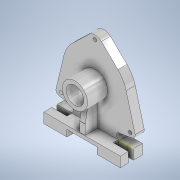
# Autodesk Inventor part: COMPRESSOR 1
Saved by Autodesk Inventor 2022 (Build 260153000, 153)
## iProperties
Created: 2023-06-16
Part Number: COMPRESSOR 1
Material: Aluminum 6061-AHC
Document SubType Name: Modeling
Designer: SENAI
Density: 2.7 g/cm^3
Appearance: Aluminum - Dark
Author: SENAI
Autodesk Inventor part; units mm, degrees
ref_plane "YZ Plane" through (0, 0, 0) normal (1, 0, 0) x (0, 1, 0)
ref_plane "XZ Plane" through (0, 0, 0) normal (0, 1, 0) x (-1, 0, 0)
ref_plane "XY Plane" through (0, 0, 0) normal (0, 0, 1) x (1, 0, 0)
sketch "Sketch1" plane through (0, 0, 0) normal (0, 0, 1) x (1, 0, 0)
  line L0 (0, 0) -> (46, 0)
  line L1 (46, 0) -> (46, 13)
  line L2 (46, 13) -> (106, 13)
  line L3 (106, 13) -> (106, 0)
  line L4 (106, 0) -> (152, 0)
  line L5 (152, 0) -> (152, 20)
  line L6 (152, 20) -> (119, 20)
  line L7 (119, 20) -> (119, 32)
  line L8 (0, 0) -> (0, 20)
  line L9 (0, 20) -> (33, 20)
  line L10 (33, 20) -> (33, 32)
  arc A0 (88.5182, 172.6658) -> (60.9434, 169.5955) centre (76, 159.7315) ccw
  line L11 (88.5182, 172.6658) -> (121.3723, 140.8686)
  arc A1 (-1.0837, 48.545) -> (6.2613, 36.9223) centre (6.0476, 44.9195) ccw
  arc A2 (149, 37.0296) -> (155.0632, 47.9932) centre (147.6772, 44.9195) ccw
  line L12 (60.9434, 169.5955) -> (30.6277, 140.8686)
  line L13 (33, 32) -> (3, 37.5227)
  line L14 (119, 32) -> (149, 37.0296)
  line L15 (155.6101, 45.954) -> (137.729, 112.6291)
  line L16 (-1.9524, 44.9195) -> (14.271, 112.6291)
  arc A3 (137.9006, 111.9892) -> (119.6299, 142.555) centre (76, 95.7315) ccw
  arc A4 (33.3683, 143.4655) -> (13.316, 108.6436) centre (76, 95.7315) ccw
  point P0 (76, 13)
  dimension "d5" = 46
  dimension "d6" = 13
  dimension "d7" = 60
  dimension "d8" = 46
  dimension "d9" = 20
  dimension "d10" = 33
  dimension "d11" = 12
  dimension "d12" = 33
  dimension "d13" = 12
  dimension "d15" = 36
  dimension "d22" = 16
  dimension "d23" = 16
  dimension "d24" = 30
  dimension "d25" = 30
  dimension "d42" = 86
  constraints: 34 end point, 17 point on circle, 9 point on line, 7 perpendicular, 5 centre point, 2 tangent, 2 vertical, 2 vertical alignment, 1 horizontal, 1 horizontal alignment, 1 midpoint
  measures "d5" distance of L0.start L0.end
  measures "d6" distance of L0.end L1.end
  measures "d7" distance of L1.end L2.end
  measures "d8" distance of L3.end L4.end
  measures "d9" distance of L4.end L5.end
  measures "d10" distance of L5.end L6.end
  measures "d11" distance of L6.end L7.end
  measures "d12" distance of L8.end L9.end
  measures "d13" distance of L9.end L10.end
  measures "d15" diameter of A0
  measures "d22" diameter of A1
  measures "d23" diameter of A2
  measures "d24" horizontal distance of L13.end L10.end
  measures "d25" horizontal distance of L14.end L7.end
  measures "d42" distance of L6.end L9.end
extrude "Extrusion1" add sketch "Sketch1" against normal blind 18 contours L8 L9 L10 L13 A1 L16 A4 L12 A0 L11 A3 L15 A2 L14 L7 L6 L5 L4 L3 L2 L1 L0
sketch "Sketch2" plane through (46, 0, 0) normal (1, 0, 0) x (0, 0, -1)
  point P0 (0, 0)
sketch "Sketch3" plane through (0, 0, 0) normal (0, 0, 1) x (1, 0, 0)
  line L0 (119, 20) -> (152, 20) projected
  line L1 (0, 20) -> (152, 20)
  line L2 (152, 20) -> (152, 0) projected
  line L3 (152, 20) -> (152, 0)
  line L4 (152, 0) -> (106, 0) projected
  line L5 (152, 0) -> (106, 0)
  line L6 (106, 0) -> (106, 13) projected
  line L7 (106, 0) -> (106, 13)
  line L8 (106, 13) -> (46, 13) projected
  line L9 (106, 13) -> (46, 13)
  line L10 (46, 13) -> (46, 0) projected
  line L11 (46, 13) -> (46, 0)
  line L12 (46, 0) -> (0, 0) projected
  line L13 (46, 0) -> (0, 0)
  line L14 (0, 0) -> (0, 20)
  constraints: 16 end point, 5 collinear, 3 perpendicular
extrude "Extrusion2" add sketch "Sketch3" along normal blind 26
sketch "Sketch4" plane through (33, 20, 0) normal (0, 1, 0) x (1, 0, 0)
  point P0 (-33, 0)
sketch "Sketch5" plane through (152, 0, -18) normal (1, 0, 0) x (0, 0, -1)
  line L0 (0, 0) -> (-44, 0) projected
  line L1 (-28, 0) -> (-28, 20)
  line L2 (0, 20) -> (-44, 20) projected
  line L3 (-28, 20) -> (-18, 20)
  line L4 (-18, 20) -> (-18, 0)
  dimension "d32" = 16
  dimension "d33" = 10
  constraints: 6 end point, 3 point on line, 1 perpendicular
  measures "d32" distance of L0.end L1.start
  measures "d33" distance of L1.end L3.end
extrude "Extrusion3" cut sketch "Sketch5" against normal blind 30
sketch "Sketch6" plane through (0, 0, 0) normal (0, 0, 1) x (1, 0, 0)
  line L0 (119, 20) -> (152, 20) projected
  point P0 (0, 0)
fillet "Fillet1" radius 4 1 edges at (119, 32, -9)
fillet "Fillet2" radius 6 1 edges at (119, 20, -9)
sketch "Sketch7" plane through (0, 0, -18) normal (-1, 0, 0) x (0, 0, 1)
  line L0 (0, 0) -> (44, 0) projected
  line L1 (18, 0) -> (18, 20)
  line L2 (18, 20) -> (0, 20) projected
  line L3 (18, 20) -> (28, 20)
  line L4 (0, 20) -> (44, 20) projected
  line L5 (28, 20) -> (28, 0)
  dimension "d38" = 18
  dimension "d39" = 10
  constraints: 6 end point, 4 point on line, 1 perpendicular, 1 vertical
  measures "d38" distance of L1.start L0.start
  measures "d39" distance of L2.start L3.end
extrude "Extrusion4" cut sketch "Sketch7" against normal blind 30
sketch "Sketch8" plane through (0, 0, 0) normal (0, 0, 1) x (1, 0, 0)
  point P0 (0, 0)
fillet "Fillet3" radius 8 1 edges at (33, 20, -9)
fillet "Fillet4" radius 2 1 edges at (33, 32, -9)
sketch "Sketch9" plane through (0, 0, 0) normal (0, 0, 1) x (1, 0, 0)
  line L0 (46, 13) -> (106, 13) projected
  arc A0 (88.5182, 172.6658) -> (60.9434, 169.5955) centre (76, 159.7315) ccw projected
  line L1 (76, 68) -> (76, 20)
  line L2 (30, 20) -> (122, 20) projected
  line L3 (76, 20) -> (81.5, 20)
  line L4 (81.5, 20) -> (81.5, 68.6125)
  line L5 (76, 20) -> (70.5, 20)
  line L6 (70.5, 20) -> (70.5, 68.6125)
  line L7 (70.5, 68.6125) -> (81.5, 68.6125)
  point P0 (0, 0)
  point P1 (76, 13)
  point P2 (76, 13)
  point P3 (76, 13)
  point P4 (74.0081, 177.621)
  dimension "d47" = 164.621
  dimension "d49" = 5.5
  dimension "d50" = 5.5
  dimension "d51" = 48
  constraints: 12 end point, 4 midpoint, 2 perpendicular, 2 point on line, 1 horizontal, 1 point on circle
  measures "d47" vertical distance of point (76, 13) point (74.008, 177.621)
  measures "d49" distance of L1.end L3.end
  measures "d50" distance of L1.end L5.end
  measures "d51" distance of L1.start L1.end
extrude "Extrusion5" add sketch "Sketch9" along normal blind 25
sketch "Sketch10" plane through (0, 0, 0) normal (0, 0, 1) x (1, 0, 0)
  circle A0 centre (76, 169.6287) radius 3.5
  circle A1 centre (145.9486, 44.6297) radius 3.5
  circle A2 centre (8.5813, 44.6297) radius 3.5
  line L0 (81.5, 68.6125) -> (70.5, 68.6125) projected
  line L1 (122.3386, 32.5597) -> (149, 37.0296) projected
  line L2 (3, 37.5227) -> (31.3621, 32.3015) projected
  point P0 (0, 0)
  point P1 (76, 68.6125)
  dimension "d55" = 7
  dimension "d56" = 7
  dimension "d57" = 7
  dimension "d78" = 8
  dimension "d79" = 8
  constraints: 3 centre point, 1 horizontal alignment, 1 midpoint
  measures "d55" diameter of A0
  measures "d56" diameter of A1
  measures "d57" diameter of A2
  measures "d78" distance from line of L1 A1.centre
  measures "d79" distance from line of L2 A2.centre
extrude "Extrusion6" cut sketch "Sketch10" against normal blind 25
sketch "Sketch11" plane through (0, 0, 0) normal (0, 0, 1) x (1, 0, 0)
  circle A0 centre (75.9727, 93.6125) radius 25
  line L0 (81.5, 68.6125) -> (70.5, 68.6125) projected
  point P0 (0, 0)
  point P1 (76, 68.6125)
  dimension "d61" = 50
  dimension "d62" = 25
  constraints: 1 centre point, 1 midpoint
  measures "d61" diameter of A0
  measures "d62" distance of point (76, 68.613) A0.centre
extrude "Extrusion7" add sketch "Sketch11" along normal blind 40
sketch "Sketch12" plane through (75.9727, 93.6125, 40) normal (0, 0, 1) x (1, 0, 0)
  circle A0 centre (0, 0) radius 17.5
  point P0 (-75.9727, -93.6125)
  dimension "d65" = 35
  constraints: 1 centre point
  measures "d65" diameter of A0
extrude "Extrusion8" cut sketch "Sketch12" against normal blind 117.25
sketch "Sketch13" plane through (81.5, 20, 0) normal (1, 0, 0) x (0, 0, -1)
  line L0 (0, 48.6125) -> (-40, 48.6125) projected
  line L1 (-20, 48.6125) -> (-25, 19.3522)
  line L2 (-25, 48.6125) -> (-25, 0) projected
  line L3 (0, 48.6125) -> (-25, 48.6125) projected
  line L4 (-20, 48.6125) -> (-25, 48.6125)
  line L5 (-25, 48.6125) -> (-25, 19.3522)
  point P0 (0, -20)
  dimension "d68" = 29.2603
  constraints: 6 end point, 1 collinear, 1 midpoint, 1 perpendicular, 1 point on line
  measures "d68" vertical distance of L1.start L1.end
extrude "Extrusion9" cut sketch "Sketch13" against normal blind 15
fillet "Fillet5" radius 4 1 edges at (76, 39.3522, 25)
sketch "Sketch14" plane through (0, 0, 0) normal (0, 0, 1) x (1, 0, 0)
  circle A0 centre (75.9727, 93.6125) radius 25 projected
  arc A1 (70.3554, 69.2518) -> (81.5123, 69.234) centre (75.9727, 93.6125) ccw
  line L0 (70.5, 68.6125) -> (70.3554, 69.2518)
  line L1 (70.4332, 69.234) -> (70.3554, 69.2518)
  line L2 (70.5, 68.6125) -> (75.9727, 68.6125) projected
  line L3 (70.5, 68.6125) -> (75.9727, 68.6125)
  line L4 (70.5, 68.6125) -> (75.9727, 68.6125)
  point P0 (0, 0)
  point P1 (70.4277, 68.9321)
  dimension "d72" = 25.2956
  constraints: 8 end point, 7 point on circle, 1 centre point, 1 collinear, 1 midpoint, 1 tangent
  measures "d72" distance of A0.centre point (70.428, 68.932)
extrude "Extrusion10" add sketch "Sketch14" along normal blind 20 contours A0 L2 L0
sketch "Sketch15" plane through (0, 0, 0) normal (0, 0, 1) x (1, 0, 0)
  line L0 (81.5, 68.6125) -> (81.5, 39.6866) projected
  line L1 (81.5, 68.6125) -> (81.5901, 69.2518)
  arc A0 (75.9727, 68.6125) -> (70.3554, 69.2518) centre (75.9727, 93.6125) ccw projected
  line L2 (75.9727, 68.6125) -> (81.5, 68.6125) projected
  arc A1 (75.9727, 68.6125) -> (81.5901, 69.2518) centre (75.9727, 93.6125) ccw
  line L3 (81.5, 68.6125) -> (75.9727, 68.6125)
  point P0 (0, 0)
  point P1 (81.545, 68.9321)
  dimension "d75" = 0.3196
  constraints: 4 end point, 3 point on circle, 1 centre point, 1 collinear, 1 concentric, 1 midpoint, 1 tangent
  measures "d75" distance from line of L2 point (81.545, 68.932)
extrude "Extrusion11" add sketch "Sketch15" along normal blind 20
body "Solid1"
